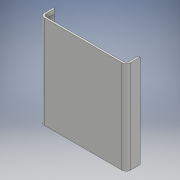
# Autodesk Inventor part: case-bottom
Saved by Autodesk Inventor 2017 (Build 210142000, 142)
## iProperties
Created: 2020-10-01
Part Number: case-bottom
Material: Generic
Document SubType Name: Modeling
Designer: jferner
Density: 1 g/cm^3
Appearance: Default
fillet2: 5.000 mm
thickness2: 2.000 mm
caseBottomWidth2: 100.000 mm
caseBottomHeight2: 16.000 mm
caseBottomDepth2: 108.000 mm
frontBackOffset2: -5.000 mm
filletInner2: 3.000 mm
filletMid2: 4.000 mm
Author: jferner
Autodesk Inventor part; units mm, degrees
ref_plane "YZ Plane" through (0, 0, 0) normal (1, 0, 0) x (0, 1, 0)
ref_plane "XZ Plane" through (0, 0, 0) normal (0, 1, 0) x (-1, 0, 0)
ref_plane "XY Plane" through (0, 0, 0) normal (0, 0, 1) x (1, 0, 0)
sketch "Sketch1" plane through (0, 0, 0) normal (0, 0, 1) x (1, 0, 0)
  line L0 (0, 16) -> (0, 5)
  line L1 (5, 0) -> (95, 0)
  line L2 (100, 5) -> (100, 16)
  arc A0 (0, 5) -> (5, 0) centre (5, 5) ccw
  arc A1 (95, 0) -> (100, 5) centre (95, 5) ccw
  line L3 (2, 16) -> (2, 5)
  arc A2 (2, 5) -> (5, 2) centre (5, 5) ccw
  line L4 (5, 2) -> (95, 2)
  arc A3 (95, 2) -> (98, 5) centre (95, 5) ccw
  line L5 (98, 5) -> (98, 16)
  line L6 (0, 16) -> (2, 16)
  line L7 (98, 16) -> (100, 16)
  point P0 (0, 0)
  dimension "fillet2" = 5
  dimension "thickness2" = 2
  dimension "caseBottomWidth2" = 100
  dimension "caseBottomHeight2" = 16
  constraints: 16 end point, 8 point on circle, 4 centre point, 4 perpendicular, 4 tangent, 2 collinear, 2 point on line, 1 equal radius, 1 horizontal, 1 vertical, 4 other
  measures "fillet2" radius of A0
  measures "thickness2" distance between parallel lines of L0 L3
  measures "caseBottomWidth2" distance between parallel lines of L2 L0
  measures "caseBottomHeight2" distance between parallel lines of L6 L1
extrude "Extrusion1" add sketch "Sketch1" along normal blind 108
ref_plane "Work Plane1" through (0, 0, 103) normal (0, 0, 1) x (1, 0, 0)
sketch "Sketch3" plane through (0, 0, 103) normal (0, 0, 1) x (1, 0, 0)
  line L0 (2, 16) -> (1, 16)
  line L1 (2, 16) -> (2, 5)
  line L2 (1, 16) -> (1, 5)
  line L3 (95, 2) -> (5, 2) projected
  line L4 (95, 2) -> (5, 2)
  line L5 (98, 16) -> (98, 5) projected
  line L6 (98, 16) -> (98, 5)
  line L7 (98, 16) -> (99, 16)
  line L8 (99, 16) -> (99, 5)
  line L9 (5, 1) -> (95, 1)
  arc A0 (2, 5) -> (5, 2) centre (5, 5) ccw
  arc A1 (95, 2) -> (98, 5) centre (95, 5) ccw
  arc A2 (1, 5) -> (5, 1) centre (5, 5) ccw
  arc A3 (95, 1) -> (99, 5) centre (95, 5) ccw
  point P0 (0, 0)
  dimension "d8" = 1
  dimension "d9" = 1
  dimension "d10" = 1
  dimension "filletInner2" = 3
  dimension "filletMid2" = 4
  constraints: 16 end point, 8 point on circle, 8 tangent, 4 centre point, 4 horizontal, 3 vertical, 2 equal radius, 1 collinear, 1 parallel
  measures "d8" distance of L0.start L0.end
  measures "d9" distance of L5.start L7.end
  measures "d10" distance between parallel lines of L9 L4
  measures "filletInner2" radius of A0
  measures "filletMid2" radius of A2
extrude "Extrusion2" cut sketch "Sketch3" against normal blind 2
ref_plane "Work Plane2" through (0, 0, 5) normal (0, 0, -1) x (-1, 0, 0)
sketch "Sketch5" plane through (0, 0, 5) normal (0, 0, -1) x (-1, 0, 0)
  line L0 (-100, 16) -> (-98, 16) projected
  line L1 (-98, 16) -> (-98, 5)
  line L2 (-99, 16) -> (-99, 5)
  line L3 (-2, 5) -> (-2, 16) projected
  line L4 (-2, 16) -> (-2, 5)
  line L5 (-2, 16) -> (0, 16) projected
  line L6 (-1, 16) -> (-1, 5)
  line L7 (-95, 2) -> (-5, 2)
  line L8 (-95, 1) -> (-5, 1)
  line L9 (-95, 2) -> (-5, 2) projected
  arc A0 (-98, 5) -> (-95, 2) centre (-95, 5) ccw
  arc A1 (-5, 2) -> (-2, 5) centre (-5, 5) ccw
  arc A2 (-99, 5) -> (-95, 1) centre (-95, 5) ccw
  arc A3 (-5, 1) -> (-1, 5) centre (-5, 5) ccw
  point P0 (0, 0)
  dimension "d21" = 1
  dimension "d22" = 3
  dimension "d23" = 4
  constraints: 12 end point, 8 point on circle, 8 tangent, 4 centre point, 4 vertical, 2 equal radius, 2 horizontal, 2 midpoint, 1 collinear
  measures "d21" distance between parallel lines of L7 L8
  measures "d22" radius of A0
  measures "d23" radius of A2
extrude "Extrusion4" cut sketch "Sketch5" against normal blind 2
sketch "Sketch7" plane through (0, 0, 108) normal (0, 0, 1) x (1, 0, 0)
  line L0 (2, 16) -> (0, 16) projected
  line L1 (2, 16) -> (1, 16)
  line L2 (1, 16) -> (1, 15)
  line L3 (1, 15) -> (2, 15)
  line L4 (2, 15) -> (2, 16)
  line L5 (99, 5) -> (99, 16) projected
  line L6 (98, 16) -> (98, 5) projected
  line L7 (99, 16) -> (98, 16)
  line L8 (98, 16) -> (98, 15)
  line L9 (98, 15) -> (99, 15)
  line L10 (99, 15) -> (99, 16)
  point P0 (0, 0)
  dimension "d28" = 1
  dimension "d29" = 1
  constraints: 16 end point, 4 parallel, 2 horizontal, 2 perpendicular, 1 collinear, 1 point on line
  measures "d28" distance between parallel lines of L0 L3
  measures "d29" distance between parallel lines of L4 L2
extrude "Extrusion6" cut sketch "Sketch7" against normal through all
equation "\"fillet2\" = fillet"
equation "\"thickness2\" = thickness"
equation "\"caseBottomWidth2\" = caseBottomWidth"
equation "\"caseBottomHeight2\" = caseBottomHeight"
equation "\"caseBottomDepth2\" = caseBottomDepth"
equation "\"d8\" = 0.5 * thickness2"
equation "\"d9\" = 0.5 * thickness2"
equation "\"d10\" = 0.5 * thickness2"
equation "\"filletInner2\" = filletInner"
equation "\"filletMid2\" = filletMid"
equation "\"d13\" = thickness2"
equation "\"d21\" = 0.5 * thickness2"
equation "\"d22\" = filletInner2"
equation "\"d23\" = filletMid2"
equation "\"d24\" = thickness2"
equation "\"d28\" = lipHeight"
equation "\"d29\" = 0.5 * thickness"
equation "\"frontBackOffset2\" = frontBackOffset"
equation "\"d15\" = frontBackOffset2"
equation "\"fillet\" = 5"
equation "\"thickness\" = 2"
equation "\"caseBottomWidth\" = 100"
equation "\"caseBottomHeight\" = 16"
equation "\"caseBottomDepth\" = 108"
equation "\"filletInner\" = 3"
equation "\"filletMid\" = 4"
equation "\"lipHeight\" = 1"
equation "\"frontBackOffset\" = -5"
body "Solid1"
